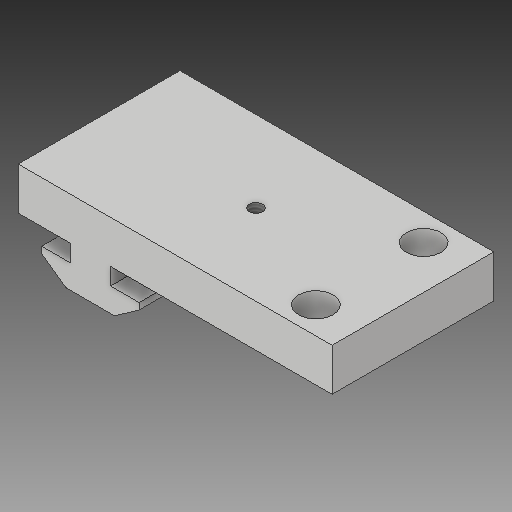
# Autodesk Inventor part: Sliderfor2020
Saved by Autodesk Inventor 2017 (Build 210142000, 142)
## iProperties
Created: 2017-12-08
Part Number: Sliderfor2020
Material: Generic
Document SubType Name: Modeling
Designer: User
Density: 1 g/cm^3
Appearance: Default
Author: User
Autodesk Inventor part; units mm, degrees
ref_plane "YZ Plane" through (0, 0, 0) normal (1, 0, 0) x (0, 1, 0)
ref_plane "XZ Plane" through (0, 0, 0) normal (0, 1, 0) x (-1, 0, 0)
ref_plane "XY Plane" through (0, 0, 0) normal (0, 0, 1) x (1, 0, 0)
sketch "Sketch1" plane through (0, 0, 0) normal (0, 0, 1) x (1, 0, 0)
  line L0 (0, 0) -> (14.5304, 0)
  line L1 (-8.7854, 6.6412) -> (8.2146, 6.6412)
  line L2 (8.2146, 1.6412) -> (2.0946, 1.6412)
  line L3 (2.0946, 1.6412) -> (2.0946, -0.3588)
  line L4 (2.0946, -0.3588) -> (5.4596, -0.3588)
  line L5 (2.5721, -3.1588) -> (-3.1429, -3.1588)
  line L6 (-3.1429, -3.1588) -> (-6.0304, -1.1208)
  line L7 (-6.0304, -1.1208) -> (-6.0304, -0.3588)
  line L8 (-6.0304, -0.3588) -> (-2.6654, -0.3588)
  line L9 (-2.6654, -0.3588) -> (-2.6654, 1.6412)
  line L10 (-2.6654, 1.6412) -> (-8.7854, 1.6412)
  line L11 (-8.7854, 1.6412) -> (-8.7854, 6.6412)
  line L12 (5.4596, -0.3588) -> (5.4596, -1.1208)
  line L13 (5.4596, -1.1208) -> (2.5721, -3.1588)
  line L14 (8.2146, 6.6412) -> (28.1746, 6.6412)
  line L15 (28.1746, 6.6412) -> (28.1746, 1.6412)
  line L16 (28.1746, 1.6412) -> (8.2146, 1.6412)
  dimension "d2" = 5
  dimension "d3" = 2
  dimension "d4" = 4.76
  dimension "d6" = 11.49
  dimension "d7" = 2.755
  dimension "d8" = 5.715
  dimension "d9" = 5.6425
  dimension "d10" = 6.12
  dimension "d11" = 0.762
  dimension "d12" = 0.762
  dimension "d16" = 26.08
  dimension "d50" = 144.786
  dimension "d51" = 2.8875
  constraints: 34 end point, 6 perpendicular, 4 point on line, 3 horizontal, 1 collinear, 1 vertical
  measures "d2" distance between parallel lines of L10 L1
  measures "d3" distance between parallel lines of L8 L10
  measures "d4" distance between parallel lines of L3 L9
  measures "d6" distance between parallel lines of L7 L12
  measures "d7" distance between parallel lines of L7 L11
  measures "d8" distance of L5.start L5.end
  measures "d9" distance from line of L5.end L11
  measures "d10" distance between parallel lines of L11 L9
  measures "d11" distance of L6.end L7.end
  measures "d12" distance of L4.end L12.end
  measures "d16" distance between parallel lines of L15 L3
  measures "d50" angle of L13 L5
  measures "d51" distance from line of L5.start L12
extrude "Extrusion1" add sketch "Sketch1" along normal blind 19.05
sketch "Sketch2" plane through (2.0946, 1.6412, 0) normal (0, -1, 0) x (1, 0, 0)
  line L0 (3.365, 0) -> (3.365, 19.05) projected
  line L1 (-8.125, 0) -> (-8.125, 19.05) projected
  line L2 (-10.88, 0) -> (-10.88, 19.05) projected
  line L3 (0, 19.05) -> (26.08, 19.05) projected
  line L4 (26.08, 0) -> (0, 0) projected
  circle A0 centre (16.1112, 11.8419) radius 1.5
  circle A1 centre (16.1112, 7.2081) radius 1.5
  point P0 (-2.0946, 0)
  dimension "d19" = 12.7462
  dimension "d20" = 12.7462
  dimension "d21" = 7.2081
  dimension "d22" = 7.2081
  dimension "d23" = 3
  dimension "d24" = 3
  constraints: 2 centre point, 2 coincident
  measures "d19" distance from line of L0 point (16.111, 11.842)
  measures "d20" distance from line of L0 point (16.111, 7.208)
  measures "d21" distance from line of point (16.111, 11.842) L3
  measures "d22" distance from line of L4 point (16.111, 7.208)
  measures "d23" diameter of A0
  measures "d24" diameter of A1
extrude "Extrusion2" cut sketch "Sketch2" against normal blind 3
sketch "Sketch3" plane through (-8.7854, 6.6412, 0) normal (0, 1, 0) x (1, 0, 0)
  line L0 (36.96, 0) -> (36.96, -19.05) projected
  line L1 (0, 0) -> (36.96, 0) projected
  line L2 (36.96, -19.05) -> (0, -19.05) projected
  point P0 (8.7854, 0)
  point P1 (31.88, -15.875)
  point P2 (31.88, -3.175)
  dimension "d27" = 5.08
  dimension "d28" = 5.08
  dimension "d36" = 3.175
  dimension "d37" = 3.175
  measures "d27" distance from line of L0 point (31.88, -3.175)
  measures "d28" distance from line of L0 point (31.88, -15.875)
  measures "d36" distance from line of L1 point (31.88, -3.175)
  measures "d37" distance from line of L2 point (31.88, -15.875)
hole "Hole1" at (23.0946, 6.6412, 15.875) at (23.0946, 6.6412, 3.175) direction (0, -1, 0) diameter 4.064 depth 25.4 tip angle 118
sketch "Sketch4" plane through (-8.7854, 6.6412, 0) normal (0, 1, 0) x (1, 0, 0)
  line L0 (36.96, -19.05) -> (0, -19.05) projected
  line L1 (0, 0) -> (36.96, 0) projected
  line L2 (36.96, 0) -> (36.96, -19.05) projected
  line L3 (0, 0) -> (0, -19.05) projected
  circle A0 centre (18.4815, -9.525) radius 1.5
  point P0 (8.7854, 0)
  dimension "d38" = 19.05
  dimension "d39" = 36.957
  dimension "d40" = 9.525
  dimension "d41" = 18.4785
  dimension "d42" = 3
  constraints: 1 centre point, 1 coincident
  measures "d38" distance between parallel lines of L0 L1
  measures "d40" distance from line of L1 point (18.482, -9.525)
  measures "d41" distance from line of L2 point (18.482, -9.525)
  measures "d42" diameter of A0
hole "Hole2" at (9.6961, 6.6412, 9.525) direction (0, -1, 0) diameter 1.5748 end through all
equation "\"d7\" = -0.5 * d6 + 0.5 * d0"
equation "\"d9\" = -0.5 * d8 + 0.5 * d0"
equation "\"d10\" = -0.5 * d4 + 0.5 * d0"
equation "\"d12\" = d11"
equation "\"d37\" = d36"
equation "\"d40\" = 0.5 * d38"
equation "\"d41\" = 0.5 * d39"
equation "\"d0\" = 17"
body "Solid1"
